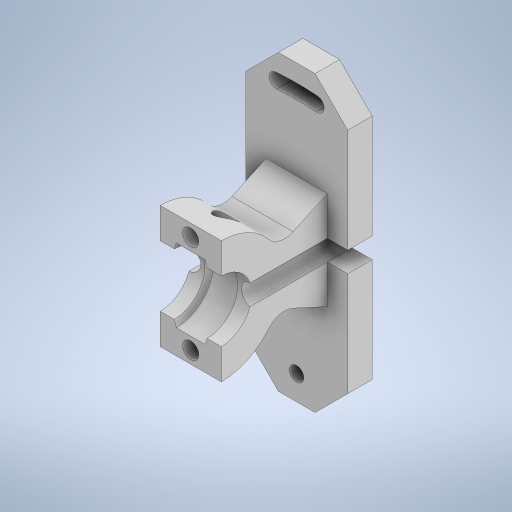
# Autodesk Inventor part: LensHolder
Saved by Autodesk Inventor 2023.1 (Build 271208000, 208)
## iProperties
Created: 2023-06-07
Part Number: LensHolder
Material: Generic
Document SubType Name: Modeling
Designer: hello
Density: 1 g/cm^3
Appearance: Default
Author: hello
Autodesk Inventor part; units mm, degrees
ref_plane "YZ Plane" through (0, 0, 0) normal (1, 0, 0) x (0, 1, 0)
ref_plane "XZ Plane" through (0, 0, 0) normal (0, 1, 0) x (-1, 0, 0)
ref_plane "XY Plane" through (0, 0, 0) normal (0, 0, 1) x (1, 0, 0)
sketch "Sketch1" plane through (0, 0, 0) normal (1, 0, 0) x (0, 1, 0)
  line L0 (-36, 0) -> (36, 0)
  line L1 (36, 0) -> (36, 6)
  line L2 (36, 6) -> (-36, 6)
  line L3 (-36, 6) -> (-36, 0)
  circle A0 centre (0, 32) radius 9
  circle A1 centre (0, 32) radius 15
  line L4 (0, 32) -> (3.7715, 23.8284) construction
  line L5 (6.2859, 18.3806) -> (12, 6)
  line L6 (0, 32) -> (-3.7715, 23.8284) construction
  line L7 (-6.2859, 18.3806) -> (-12, 6)
  line L8 (15, 32) -> (9, 32)
  line L9 (-9, 32) -> (-15, 32)
  point P0 (0, 0)
  point P1 (0, 0)
  point P2 (12, 32)
  dimension "d3" = 18
  dimension "d4" = 32
  dimension "d5" = 6
  dimension "d6" = 72
  dimension "d7" = 6
  dimension "d44" = 12
  dimension "d45" = 12
  constraints: 20 end point, 8 point on circle, 4 point on line, 2 centre point, 2 collinear, 2 horizontal, 2 midpoint, 2 parallel, 1 coincident, 1 horizontal alignment, 1 perpendicular, 1 vertical alignment
  measures "d3" diameter of A0
  measures "d4" distance of point (0, 0) L4.start
  measures "d5" distance of L0.end L1.end
  measures "d6" distance of L0.start L0.end
  measures "d7" radial gap between concentric circles of A0 A1
  measures "d44" horizontal distance of L7.end point (0, 0)
  measures "d45" horizontal distance of L5.end point (0, 0)
extrude "Extrusion1" add sketch "Sketch1" along normal mid plane 7 contours L3 L2 L1 L0 | L7 A1 L5 L2 | A1 L9 A0 L8 picked at (12.871, 30.8714)
sketch "Sketch2" plane through (3.5, 0, 0) normal (1, 0, 0) x (0, 0, -1)
  line L0 (-6, 36) -> (-6, 12) projected
  line L1 (-6, 12) -> (-18.3806, 6.2859) projected
  arc A0 (-18.3806, 6.2859) -> (-32, 15) centre (-32, 0) ccw projected
  line L2 (-32, 15) -> (-32, 9) projected
  arc A1 (-32, -9) -> (-32, 9) centre (-32, 0) ccw projected
  line L3 (-32, -9) -> (-32, -15) projected
  arc A2 (-32, -15) -> (-18.3806, -6.2859) centre (-32, 0) ccw projected
  line L4 (-18.3806, -6.2859) -> (-6, -12) projected
  line L5 (-6, -12) -> (-6, -36) projected
  line L6 (-6, -36) -> (0, -36) projected
  line L7 (0, -36) -> (0, 36) projected
  line L8 (0, 36) -> (-6, 36) projected
  arc A3 (-32, -7.5) -> (-32, 7.5) centre (-32, 0) ccw
  line L9 (-32, 9) -> (-32, 7.5)
  line L10 (-32, -9) -> (-32, -15) projected
  line L11 (-32, -7.5) -> (-32, -9)
  point P0 (0, 0)
  dimension "d14" = 1.5
  constraints: 4 end point, 2 point on circle, 2 vertical, 1 centre point, 1 coincident
  measures "d14" radial gap between concentric circles of A1 A3
extrude "Extrusion2" add sketch "Sketch2" along normal blind 4
sketch "Sketch3" plane through (-3.5, 0, 0) normal (-1, 0, 0) x (0, 0, 1)
  arc A0 (18.3806, -6.2859) -> (32, -15) centre (32, 0) ccw projected
  line L0 (18.3806, -6.2859) -> (6, -12) projected
  line L1 (6, -12) -> (6, -36) projected
  line L2 (6, -36) -> (0, -36) projected
  line L3 (0, -36) -> (0, 36) projected
  line L4 (0, 36) -> (6, 36) projected
  line L5 (6, 36) -> (6, 12) projected
  line L6 (6, 12) -> (18.3806, 6.2859) projected
  arc A1 (32, 15) -> (18.3806, 6.2859) centre (32, 0) ccw projected
  line L7 (32, 15) -> (32, 7.5) projected
  arc A2 (32, 7.5) -> (32, -7.5) centre (32, 0) ccw projected
  line L8 (32, -7.5) -> (32, -15) projected
  point P0 (0, 0)
extrude "Extrusion3" add sketch "Sketch3" along normal blind 4
sketch "Sketch4" plane through (7.5, -36, 0) normal (0, 0, -1) x (-1, 0, 0)
  line L0 (15, 72) -> (15, 0) projected
  line L1 (0, 0) -> (0, 72) projected
  line L2 (15, 0) -> (20, 0)
  line L3 (20, 0) -> (20, 72)
  line L4 (20, 72) -> (15, 72)
  line L5 (15, 72) -> (15, 0)
  line L6 (0, 0) -> (-5, 0)
  line L7 (-5, 0) -> (-5, 72)
  line L8 (-5, 72) -> (0, 72)
  line L9 (0, 72) -> (0, 0)
  point P0 (7.5, 36)
  dimension "d17" = 25
  constraints: 16 end point, 4 parallel, 2 horizontal, 2 perpendicular, 1 collinear
  measures "d17" distance of L7.end L3.end
extrude "Extrusion4" add sketch "Sketch4" against normal up to surface (6 mm away)
sketch "Sketch5" plane through (3.5, -9, 32) normal (0, 0, 1) x (1, 0, 0)
  line L0 (4, 9) -> (-11, 9)
  line L1 (-11, 9) -> (-31, 9) construction
  line L2 (-11, 1.5) -> (-11, 16.5) projected
  line L3 (-11, 11.5) -> (-31, 11.5)
  line L4 (-31, 6.5) -> (-11, 6.5)
  arc A0 (-11, 6.5) -> (-11, 11.5) centre (-11, 9) ccw
  arc A1 (-31, 11.5) -> (-31, 6.5) centre (-31, 9) ccw
  line L5 (4, 9) -> (24, 9) construction
  line L6 (4, 11.5) -> (24, 11.5)
  line L7 (24, 6.5) -> (4, 6.5)
  arc A2 (4, 11.5) -> (4, 6.5) centre (4, 9) ccw
  arc A3 (24, 6.5) -> (24, 11.5) centre (24, 9) ccw
  point P0 (-3.5, 9)
  point P1 (-3.5, 9)
  point P2 (-21, 9)
  point P3 (14, 9)
  dimension "d20" = 15
  dimension "d52" = 20
  dimension "d53" = 20
  dimension "d54" = 5
  constraints: 18 end point, 8 point on circle, 8 tangent, 4 centre point, 3 coincident, 3 midpoint, 2 parallel, 1 equal radius, 1 horizontal, 1 perpendicular, 1 point on line
  measures "d20" distance of L0.start L0.end
  measures "d52" distance of L1.start L1.end
  measures "d53" distance of L5.start L5.end
  measures "d54" distance between parallel lines of L3 L4
sketch "Sketch8" plane through (3.5, -9, 32) normal (0, 0, 1) x (1, 0, 0)
  line L0 (-11, -6) -> (4, -6) projected
  line L1 (4, 1.5) -> (4, -6) projected
  line L2 (0, 1.5) -> (4, 1.5) projected
  line L3 (0, 1.5) -> (0, 0) projected
  line L4 (-7, 0) -> (0, 0) projected
  line L5 (-7, 0) -> (-7, 1.5) projected
  line L6 (-7, 1.5) -> (-11, 1.5) projected
  line L7 (-11, -6) -> (-11, 1.5) projected
  line L8 (-7, 18) -> (0, 18) projected
  line L9 (0, 18) -> (0, 16.5) projected
  line L10 (0, 16.5) -> (4, 16.5) projected
  line L11 (4, 24) -> (4, 16.5) projected
  line L12 (-11, 24) -> (4, 24) projected
  line L13 (-11, 16.5) -> (-11, 24) projected
  line L14 (-7, 16.5) -> (-11, 16.5) projected
  line L15 (-7, 16.5) -> (-7, 18) projected
  line L16 (-7, 0) -> (0, 0) projected
  line L17 (-3.5, 0) -> (-3.5, -6)
  line L18 (-7, 18) -> (0, 18) projected
  line L19 (-3.5, 18) -> (-3.5, 24)
  line L20 (-11, 24) -> (4, 24) projected
  line L21 (-16, -27) -> (9, -27) projected
  line L22 (-16, 45) -> (9, 45) projected
  point P0 (-3.5, 9)
  point P1 (-3.5, -3)
  point P2 (-3.5, 21)
  constraints: 6 midpoint, 4 end point
hole "Hole2" at (0, -12, 32) at (0, 12, 32) direction (0, 0, -1) diameter 4 depth 16
sketch "Sketch6" plane through (3.5, -9, 32) normal (0, 0, 1) x (1, 0, 0)
  line L0 (-11, -6) -> (4, -6) projected
  line L1 (4, 1.5) -> (4, -6) projected
  line L2 (0, 1.5) -> (4, 1.5) construction
  line L3 (0, 1.5) -> (0, 0) projected
  line L4 (-7, 0) -> (0, 0) projected
  line L5 (-7, 0) -> (-7, 1.5) projected
  line L6 (-7, 1.5) -> (-11, 1.5) construction
  line L7 (-11, -6) -> (-11, 1.5) projected
  line L8 (9, 45) -> (9, -27) projected
  line L9 (9, 9) -> (-16, 9)
  line L10 (-16, -27) -> (-16, 45) projected
  line L11 (-7, 18) -> (0, 18) projected
  line L12 (0, 18) -> (0, 16.5) projected
  line L13 (0, 16.5) -> (4, 16.5) projected
  line L14 (4, 24) -> (4, 16.5) projected
  line L15 (-11, 24) -> (4, 24) projected
  line L16 (-11, 16.5) -> (-11, 24) projected
  line L17 (-7, 16.5) -> (-11, 16.5) projected
  line L18 (-7, 16.5) -> (-7, 18) projected
  line L19 (0, 1.5) -> (4, 1.5) projected
  line L20 (0, 16.5) -> (0, 1.5) projected
  line L21 (-7, 1.5) -> (-7, 16.5) projected
  line L22 (-7, 1.5) -> (-11, 1.5) projected
  arc A0 (0, 0) -> (0, 18) centre (-23.3238, 9) ccw
  arc A1 (-7, 18) -> (-7, 0) centre (16.3238, 9) ccw
  point P0 (-3.5, 9)
  point P1 (-7, 9)
  point P2 (-8.6762, 9)
  point P3 (1.6762, 9)
  point P4 (0, 9)
  dimension "d30" = 25
  dimension "d31" = 25
  constraints: 4 point on circle, 2 centre point, 2 end point, 2 midpoint
  measures "d30" radius of A0
  measures "d31" radius of A1
revolve "Revolution1" cut sketch "Sketch6" angle 360 about axis through (12.5, 0, 32) along (-1, 0, 0) contours A1 L9 L21 L22 | L22 L5 A1 | A0 L3 L19 | L19 L20 L9 A0
fillet "Fillet1" radius 5 2 edges at (0, 6.2859, 18.3806) (0, -6.2859, 18.3806)
sketch "Sketch10" plane through (-12.5, 36, 6) normal (0, 0, 1) x (1, 0, 0)
  line L0 (12.5, -66) -> (12.5, -6)
  line L1 (0, 0) -> (25, 0) projected
  circle A0 centre (12.5, -66) radius 1.75
  arc A1 (17.5, -6.2087) -> (7.5, -6.2087) centre (12.5, -66) ccw construction
  arc A2 (17.6458, -4.4648) -> (7.3542, -4.4648) centre (12.5, -66) ccw
  arc A3 (17.3542, -7.9526) -> (7.6458, -7.9526) centre (12.5, -66) ccw
  arc A4 (17.3542, -7.9526) -> (17.6458, -4.4648) centre (17.5, -6.2087) ccw
  arc A5 (7.3542, -4.4648) -> (7.6458, -7.9526) centre (7.5, -6.2087) ccw
  point P0 (12.5, -36)
  point P1 (12.5, -36)
  dimension "d46" = 60
  dimension "d47" = 3.5
  dimension "d48" = 3.5
  dimension "d49" = 5
  constraints: 11 point on circle, 6 centre point, 4 tangent, 3 coincident, 2 end point, 1 midpoint, 1 perpendicular
  measures "d46" distance of L0.end L0.start
  measures "d47" diameter of A0
  measures "d48" diameter of A4
  measures "d49" distance from line of A1.end L0
extrude "Extrusion5" cut sketch "Sketch10" against normal through all
extrude "Extrusion6" cut sketch "Sketch5" against normal up to surface (32 mm away)
chamfer "Chamfer1" distance 8 angle 45 4 edges at (12.5, 36, 3) (-12.5, 36, 3) (12.5, -36, 3) (-12.5, -36, 3)
equation "\"d3\" = LENS_D"
equation "\"d45\" = d44"
equation "\"d10\" = LENS_L"
equation "\"d30\" = LENS_R"
equation "\"d31\" = LENS_R"
equation "\"LENS_D\" = 18"
equation "\"LENS_L\" = 7"
equation "\"LENS_R\" = 25"
body "Solid1"
